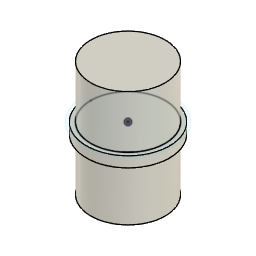
Rod Connector (Autodesk Fusion 360 design; units mm, degrees)
Autodesk Fusion 360 part; units mm, degrees
note: some values were not read from the file. Chosen so that the rebuilt part matches the saved one: which bodies a step acts on.
sketch "Sketch1" plane through (0, 0, 0) normal (0, 0, 1) x (1, 0, 0)
  circle A0 centre (0, 0) radius 14
  dimension "d1" = 28
  constraint coincident A0.centre origin
  measures "d1" diameter of A0
extrude "Extrude1" add sketch "Sketch1" along normal blind 3 draft -23 makes body 1
sketch "Sketch2" plane through (0, 0, 3) normal (0, 0, 1) x (-1, 0, 0)
  circle A0 centre (0, 0) radius 12.7266
sketch "Sketch3" plane through (0, 0, 3) normal (0, 0, 1) x (-1, 0, 0)
sketch "Sketch4" plane through (0, 0, 3) normal (0, 0, 1) x (-1, 0, 0)
  circle A0 centre (0, 0) radius 10.625
  dimension "d5" = 21.25
  constraint coincident A0.centre origin
  measures "d5" diameter of A0
extrude "Extrude2" add sketch "Sketch4" along normal blind 15 bodies 1
sketch "Sketch5" plane through (0, 0, 18) normal (0, 0, 1) x (-1, 0, 0)
  circle A0 centre (0, 0) radius 10.625
  line L0 (3.3198, -5.75) -> (6.6395, 0)
  line L1 (6.6395, 0) -> (3.3198, 5.75)
  line L2 (3.3198, 5.75) -> (-3.3198, 5.75)
  line L3 (-3.3198, 5.75) -> (-6.6395, 0)
  line L4 (-6.6395, 0) -> (-3.3198, -5.75)
  line L5 (-3.3198, -5.75) -> (3.3198, -5.75)
  dimension "d8" = 5.75
  constraint coincident A0.centre origin
  measures "d8" distance of A0.centre L5
extrude "Extrude3" cut sketch "Sketch5" against normal blind 15 contours L0 L1 L2 L3 L4 L5 bodies 1
hole "Hole1" at (-0.0502, 0.0031, 0) direction (0, 0, 1) diameter 7 depth 3 tip angle 180 bodies 1
sketch "1/4\" Bolt Hole" plane through (0, 0, 0) normal (0, 0, -1) x (1, 0, 0)
  circle A0 centre (-0.0502, -0.0031) radius 3.5
  circle A1 centre (0, 0) radius 14
split "Split1" by plane through (0, 0, 3) normal (0, 0, 1) bodies 1 makes body 2 at (-10.5722, 1.0579, 13)
cylinder "CylinderPrimitive1" add diameter 13.892 height -18 placed x (1, 0, 0) y (0, 1, 0) z (0, 0, 1) at (0, 0, 18) bodies 1 2
split "Split2" by plane through (0, 0, 3) normal (0, 0, 1) bodies 1 makes body 3 at (-10.5722, 1.0579, 13)
ref_plane "WorkPlane1" through (0, 0, 3) normal (0, 0, 1) x (-1, 0, 0)
cylinder "CylinderPrimitive2" add diameter 23.75 height -3 placed x (1, 0, 0) y (0, 1, 0) z (0, 0, 1) at (0, 0, 3) separate body makes body 4
copy_body "CopyPasteBodies1" bodies 3 makes body 5
move_body "Move1" bodies 5 to x (-1, 0, 0) y (0, 1, 0) z (0, 0, -1) at (0, 0, 3)
combine "Combine1" operation add target body 3 tool bodies 4 5 keep tools result as body 6 in component "Rod Connector"
sketch "Sketch7" plane through (0, 0, 18) normal (0, 0, 1) x (-1, 0, 0)
sketch "Sketch8" plane through (0, 0, 18) normal (0, 0, 1) x (-1, 0, 0)
component "Rod Connector" placed x (1, 0, 0) y (0, 1, 0) z (0, 0, 1) at (0, 0, 0)
hidden bodies 1
named bodies: "Body 1"
